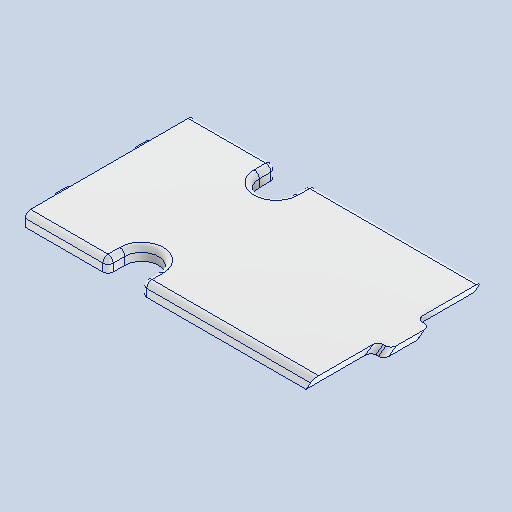
# Autodesk Inventor part: SchlittenDeckelMitte
Saved by Autodesk Inventor 2025 (Build 290162010, 162A)
## iProperties
Created: 2024-11-28
Part Number: SchlittenDeckelMitte
Material: Aluminium 6061(1)
Document SubType Name: Modeling
Designer: Admin
Density: 2.7 g/cm^3
Appearance: Aluminium - flach(1)
Author: Admin
Autodesk Inventor part; units mm, degrees
ref_plane "YZ Plane" through (0, 0, 0) normal (1, 0, 0) x (0, 1, 0)
ref_plane "XZ Plane" through (0, 0, 0) normal (0, 1, 0) x (-1, 0, 0)
ref_plane "XY Plane" through (0, 0, 0) normal (0, 0, 1) x (1, 0, 0)
sketch "Skizze1" plane through (0, 0, 0) normal (0, 0, 1) x (1, 0, 0)
  line L0 (148, 32.5) -> (-13, 32.5) projected
  line L1 (-13, -32.5) -> (148, -32.5) projected
  line L2 (57.1132, 32.5) -> (-6.5, 32.5)
  line L3 (-6.5, -32.5) -> (57.1132, -32.5)
  line L4 (57.1132, -32.5) -> (57.1132, 32.5)
  arc A0 (-13, -19.5) -> (-13, -32.5) centre (-13, -26) ccw projected
  arc A1 (-13, -32.5) -> (-13, -19.5) centre (-13, -26) ccw projected
  arc A2 (-13, 19.5) -> (-13, 32.5) centre (-13, 26) ccw projected
  arc A3 (-13, 32.5) -> (-13, 19.5) centre (-13, 26) ccw projected
  line L5 (-6.5, -32.5) -> (-6.5, -26)
  line L6 (-6.5, -26) -> (-6.5, 26)
  line L7 (-6.5, 26) -> (-6.5, 32.5)
  line L8 (-19.5, -32.5) -> (-19.5, -26)
  line L9 (-19.5, -26) -> (-19.5, 26)
  line L10 (-19.5, 26) -> (-19.5, 32.5)
  line L11 (-51.5, 32.5) -> (-51.5, -32.5)
  line L12 (-51.5, -32.5) -> (-19.5, -32.5)
  line L13 (-51.5, 32.5) -> (-19.5, 32.5)
  line L14 (57.1132, 9.5) -> (57.1132, 32.5) projected
  line L15 (57.1132, -32.5) -> (57.1132, -9.5) projected
  point P0 (57.1132, -32.2442)
  point P1 (-6.5, 32.5)
  point P2 (-16.9944, 25.4184)
  point P3 (-11.5, 13.8361)
  point P4 (-6.5242, -26.5602)
  constraints: 24 end point, 4 point on circle, 3 point on line, 2 collinear, 2 perpendicular, 1 coincident, 1 horizontal, 1 parallel, 1 vertical, 2 other
extrude "Extrusion1" add sketch "Skizze1" along normal blind 5 contours L4 L1 L5 L6 L7 L0 | L6 A1 A0 L9 A3 A2 | L9 L8 L12 L11 L13 L10
sketch "Skizze5" plane through (-51.5, -30.5, 0) normal (-1, 0, 0) x (0, 0, 1)
  line L0 (0, 43.5) -> (2.5, 43.5) projected
  line L1 (2.5, 17.5) -> (0, 17.5) projected
  line L2 (0, 43.5) -> (2.5, 43.5)
  line L3 (2.5, 43.5) -> (2.5, 48.5)
  line L4 (2.5, 48.5) -> (0, 48.5)
  line L5 (0, 48.5) -> (0, 43.5)
  line L6 (0, 17.5) -> (2.5, 17.5)
  line L7 (2.5, 17.5) -> (2.5, 12.5)
  line L8 (2.5, 12.5) -> (0, 12.5)
  line L9 (0, 12.5) -> (0, 17.5)
  point P0 (0, 30.5)
  dimension "d7" = 2.5
  dimension "d8" = 5
  dimension "d9" = 2.5
  dimension "d10" = 5
  constraints: 16 end point, 4 parallel, 2 horizontal, 2 perpendicular
  measures "d7" distance of L4.end L3.end
  measures "d8" distance of L3.end L2.end
  measures "d9" distance of L7.end L8.end
  measures "d10" distance of L6.end L7.end
extrude "Extrusion3" add sketch "Skizze5" along normal blind 3
sketch "Skizze6" plane through (0, 0, 0) normal (0, 0, -1) x (-1, 0, 0)
  line L0 (-57.1132, -32.5) -> (-57.1132, -9.5) projected
  arc A0 (-57.1132, -9.5) -> (-59.1132, -7.5) centre (-59.1132, -9.5) ccw projected
  line L1 (-59.1132, -7.5) -> (-60.1132, -7.5) projected
  arc A1 (-62.1132, -5.5) -> (-60.1132, -7.5) centre (-60.1132, -5.5) ccw projected
  line L2 (-62.1132, -5.5) -> (-62.1132, 5.5) projected
  arc A2 (-60.1132, 7.5) -> (-62.1132, 5.5) centre (-60.1132, 5.5) ccw projected
  line L3 (-60.1132, 7.5) -> (-59.1132, 7.5) projected
  arc A3 (-59.1132, 7.5) -> (-57.1132, 9.5) centre (-59.1132, 9.5) ccw projected
  line L4 (-57.1132, 9.5) -> (-57.1132, 32.5) projected
  line L5 (-57.1132, 32.5) -> (-47.1132, 32.5)
  line L6 (-57.1132, 32.5) -> (6.5, 32.5) projected
  line L7 (-47.1132, 32.5) -> (-47.1132, -32.5)
  line L8 (6.5, -32.5) -> (-57.1132, -32.5) projected
  line L9 (-47.1132, -32.5) -> (-57.1132, -32.5)
  point P0 (0, 0)
  point P1 (13, 32.5)
  point P2 (13, -32.5)
  dimension "d14" = 10
  constraints: 6 end point, 2 perpendicular, 2 point on line
  measures "d14" distance of L4.end L5.end
sketch "Skizze7" plane through (-6.5, 32.5, 0) normal (0, 1, 0) x (1, 0, 0)
  line L0 (63.6132, 0) -> (66.5, -5)
  point P0 (6.5, 0)
  constraints: 2 end point, 1 coincident, 2 other
sweep "Sweeping2" add profiles "Skizze6" path "Skizze7"
fillet "Rundung3" radius 2 15 edges at (26.75, 32.5, 5) (58.5566, -32.5, 5) (25.3066, -32.5, 5) (-6.5, 32.5, 2.5) (-19.5, 32.5, 2.5) (-13, 19.5, 5) (-6.5, 29.25, 5) (-19.5, 29.25, 5) (-35.5, 32.5, 5) (-35.5, -32.5, 5) (-13, -19.5, 5) (-6.5, -29.25, 5) (-19.5, -29.25, 5) (-19.5, -32.5, 2.5) (-6.5, -32.5, 2.5)
sketch "Skizze8" plane through (0, 0, 0) normal (0, 0, -1) x (-1, 0, 0)
  circle A0 centre (-50.6132, 26) radius 2.65 projected
  circle A1 centre (-50.6132, -26) radius 2.65 projected
  point P0 (0, 0)
extrude "Extrusion4" cut sketch "Skizze8" against normal blind 3.3
